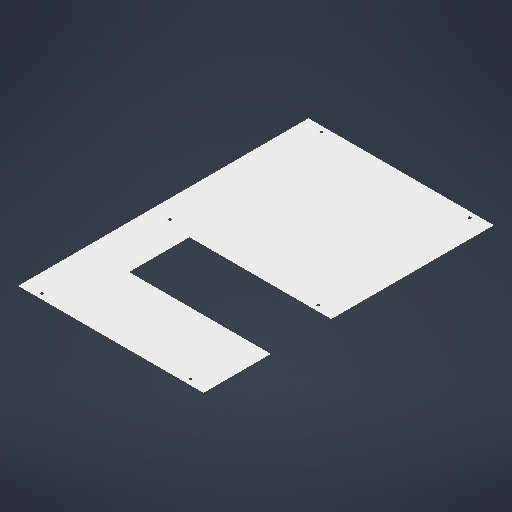
# Autodesk Inventor part: PlaqueSupperieur
Saved by Autodesk Inventor 2026.2 (Build 302298010, 298A)
## iProperties
Created: 2026-05-18
Part Number: PlaqueSupperieur
Material: Générique
Document SubType Name: Modeling
Designer: romai
Density: 1 g/cm^3
Appearance: Par défaut
Author: romai
Autodesk Inventor part; units mm, degrees
ref_plane "YZ Plane" through (0, 0, 0) normal (1, 0, 0) x (0, 1, 0)
ref_plane "XZ Plane" through (0, 0, 0) normal (0, 1, 0) x (-1, 0, 0)
ref_plane "XY Plane" through (0, 0, 0) normal (0, 0, 1) x (1, 0, 0)
sketch "Esquisse1" plane through (0, 0, 0) normal (0, 1, 0) x (-1, 0, 0)
  line L0 (235, 367.5) -> (-235, 367.5)
  line L1 (-235, 367.5) -> (-235, -367.5)
  line L2 (-235, -367.5) -> (235, -367.5)
  line L3 (235, -367.5) -> (235, 367.5)
  line L4 (235, 367.5) -> (-235, -367.5) construction
  line L5 (-235, 367.5) -> (235, -367.5) construction
  line L6 (227.0068, 355) -> (-227.0068, 355)
  line L7 (-227.0068, -355) -> (227.0068, -355)
  line L8 (227.0068, -355) -> (227.0068, 355)
  line L9 (227.0068, 355) -> (-227.0068, -355) construction
  line L10 (-227.0068, 355) -> (227.0068, -355) construction
  line L11 (122.9932, 195) -> (-227.0068, 195)
  line L12 (-227.0068, 195) -> (-227.0068, 45)
  line L13 (-227.0068, 45) -> (122.9932, 45)
  line L14 (122.9932, 45) -> (122.9932, 195)
  line L15 (122.9932, 195) -> (-227.0068, 45) construction
  line L16 (-227.0068, 195) -> (122.9932, 45) construction
  circle A0 centre (-187.0068, -352.5) radius 2.5
  circle A1 centre (187.0068, -352.5) radius 2.5
  circle A2 centre (187.0068, 30) radius 2.5
  circle A3 centre (-187.0068, 30) radius 2.5
  circle A4 centre (-187.0068, 352.5) radius 2.5
  circle A5 centre (187.0068, 352.5) radius 2.5
  line L17 (-227.0068, -355) -> (-197.0068, -355)
  line L18 (-227.0068, -325) -> (-227.0068, -355)
  line L19 (-227.0068, 45) -> (-235, 45)
  line L20 (-227.0068, 195) -> (-235, 195)
  line L21 (-227.0068, 355) -> (-227.0068, 195)
  line L22 (-227.0068, 45) -> (-227.0068, -355)
  point P0 (0, 0)
  point P1 (-52.0068, 120)
  dimension "d0" = 735
  dimension "d1" = 470
  dimension "d2" = 12.5
  dimension "d3" = 160
  dimension "d4" = 150
  dimension "d5" = 350
  dimension "d6" = 5
  dimension "d7" = 5
  dimension "d8" = 5
  dimension "d9" = 5
  dimension "d10" = 5
  dimension "d11" = 5
  dimension "d16" = 40
  dimension "d17" = 40
  dimension "d21" = 40
  dimension "d22" = 397.5
  dimension "d23" = 397.5
  constraints: 46 end point, 7 parallel, 6 centre point, 6 midpoint, 6 perpendicular, 4 horizontal, 4 tangent, 3 point on line
  measures "d0" distance of L0.end L1.end
  measures "d1" distance of L0.start L0.end
  measures "d2" distance between parallel lines of L2 L7
  measures "d3" distance between parallel lines of L6 L11
  measures "d4" distance of L13.end L11.start
  measures "d5" distance of L11.start L11.end
  measures "d6" diameter of A0
  measures "d7" diameter of A1
  measures "d8" diameter of A2
  measures "d9" diameter of A3
  measures "d10" diameter of A4
  measures "d11" diameter of A5
  measures "d16" distance from line of L8 A1.centre
  measures "d17" distance from line of L8 A5.centre
  measures "d21" distance from line of L8 A2.centre
  measures "d22" distance from line of L2 A2.centre
  measures "d23" distance from line of L2 A3.centre
extrude "Extrusion1" add sketch "Esquisse1" along normal blind 2 contours L3 L2 L1 L19 L22 L18 L7 L8 L6 L21 L20 L0 | L21 L6 L8 L7 L18 L22 L13 L14 L11
